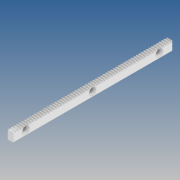
# Autodesk Inventor part: 3222_Motor Rack_V1
Saved by Autodesk Inventor 2020 (Build 240168000, 168)
## iProperties
Created: 2019-10-21
Part Number: 3222_Motor Rack_V1
Material: Acetal Resin, White
Document SubType Name: Modeling
Designer: RFLab
Density: 1.425 g/cm^3
Appearance: Smooth - White
Author: RFLab
Autodesk Inventor part; units mm, degrees
ref_plane "YZ Plane" through (0, 0, 0) normal (1, 0, 0) x (0, 1, 0)
ref_plane "XZ Plane" through (0, 0, 0) normal (0, 1, 0) x (-1, 0, 0)
ref_plane "XY Plane" through (0, 0, 0) normal (0, 0, 1) x (1, 0, 0)
sketch "Sketch1" plane through (0, 0, 0) normal (0, 0, 1) x (1, 0, 0)
  line L0 (-2, -3.5) -> (2, -3.5)
  line L1 (2, -3.5) -> (2, 3.5)
  line L2 (2, 3.5) -> (-2, 3.5)
  line L3 (-2, 3.5) -> (-2, -3.5)
  point P0 (0, 0)
  dimension "d0" = 4
  dimension "d1" = 7
  dimension "d2" = 3.5
  dimension "d3" = 2
  constraints: 8 end point, 2 parallel, 1 horizontal, 1 perpendicular
  measures "d0" distance of L0.start L0.end
  measures "d1" distance of L0.end L1.end
  measures "d2" distance from line of point (0, 0) L0
  measures "d3" distance from line of point (0, 0) L3
extrude "Extrusion1" add sketch "Sketch1" along normal blind 125
sketch "Sketch2" plane through (2, -3.5, 0) normal (1, 0, 0) x (0, 0, -1)
  line L0 (-125, 5) -> (0, 5) construction
  line L1 (0, 0) -> (0, 7) construction
  line L2 (0, 7) -> (-125, 7) construction
  line L3 (-125, 0) -> (-125, 7) construction
  line L4 (0, 0) -> (-125, 0) construction
  line L5 (0, 0) -> (0, 7) projected
  line L6 (0, 6) -> (-125, 6)
  line L7 (-125, 0) -> (-125, 7) projected
  line L8 (-0.864, 6) -> (-0.5, 7)
  line L9 (0, 7) -> (-125, 7) projected
  line L10 (-1.364, 6) -> (-1.7279, 7)
  point P0 (0, 3.5)
  dimension "d6" = 1
  dimension "d7" = 70
  dimension "d8" = 70
  dimension "d9" = 0.5
  dimension "d10" = 0.5
  constraints: 6 end point, 6 point on line, 1 horizontal
  measures "d6" distance between parallel lines of L2 L6
  measures "d7" angle of L6 L10
  measures "d8" angle of L6 L8
  measures "d9" distance of L10.start L8.start
  measures "d10" distance of L1.end L8.end
extrude "Extrusion2" cut sketch "Sketch2" against normal through all contours L6 L10 L9 L8
pattern_linear "Rectangular Pattern1" count 63 spacing 2 along (0, 0, 1) of "Extrusion2"
sketch "Sketch3" plane through (2, -3.5, 0) normal (1, 0, 0) x (0, 0, -1)
  line L0 (0, 3.5) -> (-125, 3.5)
  point P0 (-10, 3.5)
  point P1 (-115, 3.5)
  point P2 (-62.5, 3.5)
  dimension "d16" = 10
  dimension "d17" = 10
  constraints: 2 end point, 2 point on line, 1 horizontal, 1 midpoint
  measures "d16" distance of L0.start point (-10, 3.5)
  measures "d17" distance of L0.end point (-115, 3.5)
hole "Hole1" at (2, 0, 10) at (2, 0, 115) at (2, 0, 62.5) direction (-1, 0, 0) diameter 2.9 end through all countersink diameter 5.5 countersink angle 90 clearance for "Flat Head Machine Screw" size "M2.5" standard "Ansi Metric M Profile"
equation "\"d2\" = 0.5 * d1"
equation "\"d3\" = 0.5 * d0"
equation "\"d8\" = d7"
body "Solid1"
